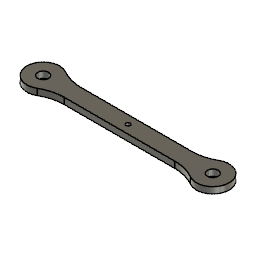
BARRA_DIRECCION_V2 (Autodesk Fusion 360 design; units mm, degrees)
Autodesk Fusion 360 part; units mm, degrees
sketch "Boceto1" plane through (0, 0, 0) normal (0, 0, 1) x (1, 0, 0)
  circle A0 centre (-40, 0) radius 2.5
  circle A1 centre (40, 0) radius 2.5
  circle A2 centre (0, 0) radius 1
  line L0 (0, 4) -> (0, -4) construction
  circle A3 centre (40, 0) radius 7.75
  circle A4 centre (-40, 0) radius 7.75
  line L1 (-33.362, 4) -> (33.362, 4)
  line L2 (-33.362, -4) -> (33.362, -4)
  line L3 (-40, 0) -> (40, 0) construction
  dimension "d1" = 5
  dimension "d4" = 80
  dimension "d5" = 5
  dimension "d6" = 2
  dimension "d9" = 15.5
  dimension "d10" = 15.5
  dimension "d12" = 4
  dimension "d13" = 4
  constraint midpoint A2.centre L0
  constraint coincident A2.centre origin
  constraint concentric A1 A3
  constraint concentric A0 A4
  constraint coincident A4 L1.start
  constraint coincident A3 L1.end
  constraint horizontal L1
  constraint coincident A4 L2.start
  constraint coincident A3 L2.end
  constraint parallel L1 L2
  constraint coincident A0.centre A4.centre
  constraint coincident A1.centre A3.centre
  constraint horizontal L3
  constraint coincident A2.centre L3
  measures "d1" diameter of A0
  measures "d4" distance of A1.centre A0.centre
  measures "d5" diameter of A1
  measures "d6" diameter of A2
  measures "d9" diameter of A3
  measures "d10" diameter of A4
  measures "d12" distance of L1 L3
  measures "d13" distance of L2 L3
extrude "Extruir1" add sketch "Boceto1" along normal blind 3 contours A3
extrude "Extruir2" add sketch "Boceto1" along normal blind 3 contours A3 A4 L1 L2 | A4
fillet "Empalme1" radius 20 1 edges at (-33.362, -4, 1.5)
fillet "Empalme2" radius 20 1 edges at (33.362, -4, 1.5)
fillet "Empalme3" radius 20 1 edges at (33.362, 4, 1.5)
fillet "Empalme4" radius 20 1 edges at (-33.362, 4, 1.5)
